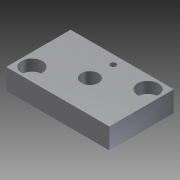
# Autodesk Inventor part: 13_0204_074
Saved by Autodesk Inventor 2014 (Build 180170000, 170)
## iProperties
Created: 2013-05-21
Part Number: 13_0204_074
Material: Allgemein
Document SubType Name: Modeling
Designer: vogel
Density: 1 g/cm^3
Appearance: Vorgabe
Author: vogel
Autodesk Inventor part; units mm, degrees
ref_plane "YZ Plane" through (0, 0, 0) normal (1, 0, 0) x (0, 1, 0)
ref_plane "XZ Plane" through (0, 0, 0) normal (0, 1, 0) x (-1, 0, 0)
ref_plane "XY Plane" through (0, 0, 0) normal (0, 0, 1) x (1, 0, 0)
sketch "Skizze1" plane through (0, 0, 0) normal (0, 0, 1) x (1, 0, 0)
  line L0 (-20, 12.5) -> (20, 12.5)
  line L1 (20, 12.5) -> (20, -12.5)
  line L2 (20, -12.5) -> (-20, -12.5)
  line L3 (-20, -12.5) -> (-20, 12.5)
  line L4 (-28, 0) -> (28, 0) projected
  line L5 (0, -17.5) -> (0, 17.5) projected
  point P0 (0, 0)
  dimension "d0" = 40
  dimension "d1" = 25
  constraints: 8 end point, 2 parallel, 1 horizontal, 1 perpendicular, 2 other
  measures "d0" distance of L0.start L0.end
  measures "d1" distance of L2.end L0.start
extrude "Extrusion1" add sketch "Skizze1" along normal blind 8
sketch "Skizze2" plane through (0, 0, 8) normal (0, 0, 1) x (1, 0, 0)
  line L0 (-28, 0) -> (28, 0) projected
  line L1 (0, -17.5) -> (0, 17.5) projected
  line L2 (-15, 7.5) -> (15, 7.5)
  line L3 (15, 7.5) -> (15, -7.5)
  line L4 (15, -7.5) -> (-15, -7.5)
  line L5 (-15, -7.5) -> (-15, 7.5)
  point P0 (0, 0)
  dimension "d4" = 15
  dimension "d5" = 30
  constraints: 8 end point, 2 coincident, 2 parallel, 1 horizontal, 1 perpendicular, 2 other
  measures "d4" distance of L4.end L2.start
  measures "d5" distance of L2.start L2.end
hole "Bohrung1" at (-15, -7.5, 8) at (15, 7.5, 8) direction (0, 0, -1) diameter 4.5 end through all counterbore diameter 8 counterbore depth 4.4
sketch "Skizze3" plane through (0, 0, 8) normal (0, 0, 1) x (1, 0, 0)
  point P0 (0, 0)
  point P1 (0, 0)
  constraints: 1 coincident
hole "Bohrung2" at (0, 0, 8) direction (0, 0, -1) diameter 3 end through all
hole "Bohrung3" at (0, 0, 0) direction (0, 0, 1) diameter 6.6 end through all countersink diameter 12.4 countersink angle 90
sketch "Skizze4" plane through (0, 0, 8) normal (0, 0, 1) x (1, 0, 0)
  line L0 (-28, 0) -> (28, 0) projected
  line L1 (0, -17.5) -> (0, 17.5) projected
  point P0 (0, 9)
  dimension "d29" = 9
  constraints: 1 point on line
  measures "d29" distance from line of point (0, 9) L0
hole "Bohrung4" at (0, 9, 8) direction (0, 0, -1) diameter 2.2 depth 5 tip angle 118
